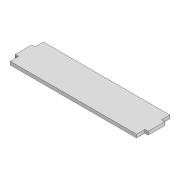
# Autodesk Inventor part: Top 1
Saved by Autodesk Inventor 2022 (Build 260153000, 153)
## iProperties
Created: 2022-06-16
Part Number: Top 1
Material: Generic
Document SubType Name: Modeling
Designer: ADMIN
Density: 1 g/cm^3
Appearance: Default
Author: ADMIN
Autodesk Inventor part; units mm, degrees
ref_plane "YZ Plane" through (0, 0, 0) normal (1, 0, 0) x (0, 1, 0)
ref_plane "XZ Plane" through (0, 0, 0) normal (0, 1, 0) x (-1, 0, 0)
ref_plane "XY Plane" through (0, 0, 0) normal (0, 0, 1) x (1, 0, 0)
sketch "Sketch1" plane through (0, 0, 0) normal (0, 1, 0) x (-1, 0, 0)
  line L0 (-82.3159, -38.8456) -> (107.6841, -38.8456)
  line L1 (107.6841, -38.8456) -> (107.6841, 11.1544)
  line L2 (107.6841, 11.1544) -> (-82.3159, 11.1544)
  line L3 (-82.3159, 11.1544) -> (-82.3159, -38.8456)
  line L4 (107.6841, -1.3456) -> (112.6841, -1.3456)
  line L5 (112.6841, -1.3456) -> (112.6841, -26.3456)
  line L6 (112.6841, -26.3456) -> (107.6841, -26.3456)
  line L7 (107.6841, -26.3456) -> (107.6841, -1.3456)
  line L8 (12.6841, 11.1544) -> (12.6841, -38.8456)
  line L9 (-82.3159, -1.3456) -> (-87.3159, -1.3456)
  line L10 (-87.3159, -1.3456) -> (-87.3159, -26.3456)
  line L11 (-87.3159, -26.3456) -> (-82.3159, -26.3456)
  point P0 (0, 0)
  dimension "d0" = 190
  dimension "d1" = 50
  dimension "d2" = 5
  dimension "d3" = 25
  dimension "d4" = 12.5
  constraints: 24 end point, 4 parallel, 4 symmetric about line, 2 horizontal, 2 midpoint, 2 perpendicular, 1 point on line
  measures "d0" distance of L0.start L0.end
  measures "d1" distance of L0.end L1.end
  measures "d2" distance of L5.end L6.end
  measures "d3" distance of L4.end L5.end
  measures "d4" distance from line of L1.end L4
extrude "Extrusion1" add sketch "Sketch1" along normal blind 5
body "Solid1"
